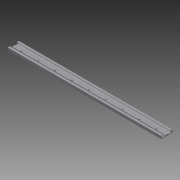
# Autodesk Inventor part: aluminum slider
Saved by Autodesk Inventor 2015 SP1 (Build 190203100, 203)
## iProperties
Created: 2015-01-14
Part Number: aluminum slider
Material: Generic
Document SubType Name: Modeling
Designer: Jarod
Density: 1 g/cm^3
Appearance: Default
Author: Jarod
Autodesk Inventor part; units mm, degrees
ref_plane "YZ Plane" through (0, 0, 0) normal (1, 0, 0) x (0, 1, 0)
ref_plane "XZ Plane" through (0, 0, 0) normal (0, 1, 0) x (-1, 0, 0)
ref_plane "XY Plane" through (0, 0, 0) normal (0, 0, 1) x (1, 0, 0)
sketch "Sketch1" plane through (0, 0, 0) normal (1, 0, 0) x (0, 1, 0)
  line L0 (0, 0) -> (0, -40.005)
  line L1 (0, -40.005) -> (9.4996, -40.005)
  line L2 (0, 0) -> (9.4996, 0)
  line L3 (9.4996, 0) -> (9.4996, -7.493)
  line L4 (9.4996, 0) -> (16.9926, 0) construction
  line L5 (9.4996, -40.005) -> (9.4996, -32.512)
  line L6 (9.4996, -40.005) -> (16.9926, -40.005) construction
  line L7 (9.4996, -7.493) -> (8.001, -7.493)
  line L8 (9.4996, -32.512) -> (8.001, -32.512)
  line L9 (9.4996, -32.512) -> (10.9982, -32.512) construction
  line L10 (8.001, -7.493) -> (8.001, -2.0066)
  line L11 (8.001, -7.493) -> (13.4874, -7.493) construction
  line L12 (8.001, -32.512) -> (8.001, -37.9984)
  line L13 (8.001, -32.512) -> (13.4874, -32.512) construction
  line L14 (8.001, -2.0066) -> (2.4892, -2.0066)
  line L15 (2.4892, -2.0066) -> (2.4892, -15.0114)
  line L16 (2.4892, -15.0114) -> (4.9784, -15.0114)
  line L17 (8.001, -37.9984) -> (2.4892, -37.9984)
  line L18 (8.001, -37.9984) -> (13.5128, -37.9984) construction
  line L19 (2.4892, -37.9984) -> (2.4892, -24.9936)
  line L20 (2.4892, -24.9936) -> (4.9784, -24.9936)
  line L21 (4.9784, -15.0114) -> (3.9878, -15.0114) construction
  line L22 (3.9878, -15.0114) -> (3.9878, -24.9936) construction
  line L23 (4.9784, -15.0114) -> (3.9878, -16.002)
  line L24 (4.9784, -15.0114) -> (6.3793, -15.0114) construction
  line L25 (4.9784, -24.9936) -> (3.9878, -24.003)
  line L26 (4.9784, -24.9936) -> (6.3793, -24.9936) construction
  line L27 (3.9878, -24.003) -> (3.9878, -16.002)
  dimension "d0" = 40.005
  dimension "d1" = 9.4996
  dimension "d2" = 9.4996
  dimension "d3" = 7.493
  dimension "d4" = 90
  dimension "d5" = 7.493
  dimension "d6" = 90
  dimension "d7" = 1.4986
  dimension "d8" = 1.4986
  dimension "d9" = 180
  dimension "d10" = 5.4864
  dimension "d11" = 90
  dimension "d12" = 5.4864
  dimension "d13" = 90
  dimension "d22" = 5.5118
  dimension "d23" = 13.0048
  dimension "d24" = 2.4892
  dimension "d25" = 90
  dimension "d26" = 5.5118
  dimension "d27" = 180
  dimension "d28" = 13.0048
  dimension "d29" = 90
  dimension "d30" = 2.4892
  dimension "d31" = 90
  dimension "d32" = 0.9906
  dimension "d33" = 135
  dimension "d34" = 135
  constraints: 56 end point, 14 horizontal, 8 equal length, 5 perpendicular, 5 vertical, 4 point on line, 1 collinear
  measures "d0" distance of L0.start L0.end
  measures "d1" distance of L0.end L1.end
  measures "d2" distance of L0.start L2.end
  measures "d3" distance of L2.end L3.end
  measures "d4" angle of L3 L4
  measures "d5" distance of L1.end L5.end
  measures "d6" angle of L6 L5
  measures "d7" distance of L3.end L7.end
  measures "d8" distance of L5.end L8.end
  measures "d9" angle of L8 L9
  measures "d10" distance of L7.end L10.end
  measures "d11" angle of L11 L10
  measures "d12" distance of L8.end L12.end
  measures "d13" angle of L12 L13
  measures "d22" distance of L10.end L14.end
  measures "d23" distance of L14.end L15.end
  measures "d24" distance of L15.end L16.end
  measures "d25" angle of L16 L15
  measures "d26" distance of L12.end L17.end
  measures "d27" angle of L17 L18
  measures "d28" distance of L17.end L19.end
  measures "d29" angle of L17 L19
  measures "d30" distance of L19.end L20.end
  measures "d31" angle of L19 L20
  measures "d32" distance of L16.end L21.end
  measures "d33" angle of L23 L24
  measures "d34" angle of L26 L25
extrude "Extrusion1" add sketch "Sketch1" along normal blind 546.1
sketch "Sketch2" plane through (0, 3.9878, -16.002) normal (0, 1, 0) x (1, 0, 0)
  line L0 (0, 8.001) -> (0, 0) projected
  line L1 (0, 0) -> (546.1, 0) projected
  line L2 (546.1, 8.001) -> (546.1, 0) projected
  line L3 (0, 8.001) -> (546.1, 8.001) projected
  point P0 (0, -16.002)
  point P1 (29.9974, 3.9878)
  dimension "d37" = 29.9974
  dimension "d38" = 3.9878
  measures "d37" distance from line of point (29.997, 3.988) L0
  measures "d38" distance from line of L1 point (29.997, 3.988)
hole "Hole1" at (29.9974, 3.9878, -19.9898) direction (0, -1, 0) diameter 3.9878 end through all countersink diameter 5.9944 countersink angle 82
pattern_linear "Rectangular Pattern1" count 9 spacing 59.9948 along (1, 0, 0) of "Hole1"
body "Solid1"
